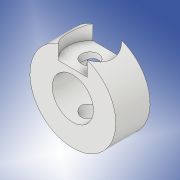
# Autodesk Inventor part: WA003.ip
Saved by Autodesk Inventor 2017 SP1 (Build 210196100, 196)
## iProperties
Created: 2017-08-01
Part Number: WA003.ip
Material: ABS Plastic
Document SubType Name: Modeling
Designer: Zach
Density: 1.06 g/cm^3
Appearance: CR White
Author: Zach
Autodesk Inventor part; units mm, degrees
ref_plane "YZ Plane" through (0, 0, 0) normal (1, 0, 0) x (0, 1, 0)
ref_plane "XY Plane" through (0, 0, 0) normal (0, 0, 1) x (1, 0, 0)
sketch "Sketch1" plane through (0, 0, 0) normal (0, 0, 1) x (1, 0, 0)
  circle A0 centre (0, 0) radius 6
  circle A1 centre (0, 0) radius 12.5
  dimension "d0" = 12
  dimension "d1" = 25
  constraints: 2 centre point, 2 coincident
  measures "d0" diameter of A0
  measures "d1" diameter of A1
extrude "Extrusion1" add sketch "Sketch1" along normal blind 10
sketch "Sketch2" plane through (0, 0, 0) normal (0, 1, 0) x (-1, 0, 0)
  circle A0 centre (0, 5) radius 2.5
  line L0 (6, 0) -> (6, 10) projected
  point P0 (0, 0)
  point P1 (6, 5)
  dimension "d4" = 5
  constraints: 1 centre point, 1 horizontal alignment, 1 midpoint, 1 vertical alignment
  measures "d4" diameter of A0
extrude "Extrusion2" cut sketch "Sketch2" along normal through all both and the other way through all
ref_plane "Work Plane1" through (0, 12.5, 0) normal (0, 1, 0) x (-1, 0, 0)
sketch "Sketch4" plane through (0, 12.5, 0) normal (0, 1, 0) x (-1, 0, 0)
  spline S0 degree 8 poles (2.5, 5) (2.5, 5.2613) (2.4688, 5.5221) (2.4066, 5.7804) (2.3127, 6.0339) (2.1861, 6.2798) (2.0251, 6.5144) (1.828, 6.7323) (1.3947, 7.0908) (1.1606, 7.2449) (0.8947, 7.3748) (0.6036, 7.4701) (0.2962, 7.5238) (-0.0173, 7.5328) (-0.3265, 7.4973) (-0.927, 7.3431) (-1.2062, 7.2245) (-1.4564, 7.0744) (-1.6765, 6.9) (-1.8664, 6.7071) (-2.0266, 6.5008) (-2.1581, 6.2854) (-2.3815, 5.8106) (-2.4663, 5.546) (-2.5169, 5.2746) (-2.5338, 5) (-2.5169, 4.7254) (-2.4663, 4.454) (-2.3815, 4.1894) (-2.1645, 3.7282) (-2.0429, 3.5262) (-1.8964, 3.3322) (-1.7241, 3.1495) (-1.5253, 2.9819) (-1.3, 2.8342) (-1.0485, 2.712) (-0.5121, 2.5377) (-0.2336, 2.4833) (0.0549, 2.4652) (0.3445, 2.486) (0.6257, 2.5448) (0.8897, 2.6372) (1.1293, 2.7558) (1.6409, 3.0804) (1.8944, 3.3103) (2.1007, 3.5658) (2.2623, 3.8384) (2.3815, 4.1219) (2.4604, 4.412) (2.5, 4.7056) (2.5, 5) knots 0 0 0 0 0 0 0 0 0 0.155158 0.155158 0.155158 0.155158 0.155158 0.155158 0.155158 0.286737 0.286737 0.286737 0.286737 0.286737 0.286737 0.286737 0.422792 0.422792 0.422792 0.422792 0.422792 0.422792 0.422792 0.579084 0.579084 0.579084 0.579084 0.579084 0.579084 0.579084 0.706752 0.706752 0.706752 0.706752 0.706752 0.706752 0.706752 0.82726 0.82726 0.82726 0.82726 0.82726 0.82726 0.82726 1 1 1 1 1 1 1 1 1 projected
  circle A0 centre (0, 5) radius 6.5
  point P0 (0, 0)
  dimension "d8" = 13
  constraints: 1 centre point, 1 horizontal alignment, 1 vertical alignment, 1 other
  measures "d8" diameter of A0
extrude "Extrusion3" cut sketch "Sketch4" against normal blind 5
body "Solid1"
